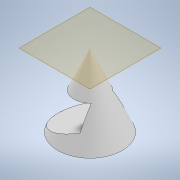
# Autodesk Inventor part: Деталь2Инди
Saved by Autodesk Inventor 2021.1 (Build 251245010, 245A)
## iProperties
Created: 2023-10-12
Part Number: Деталь2Инди
Material: Типовые
Document SubType Name: Modeling
Designer: Lenovo
Density: 1 g/cm^3
Appearance: По умолчанию
Author: Lenovo
Autodesk Inventor part; units mm, degrees
ref_plane "YZ Plane" through (0, 0, 0) normal (1, 0, 0) x (0, 1, 0)
ref_plane "XY Plane" through (0, 0, 0) normal (0, 0, 1) x (1, 0, 0)
sketch "Эскиз1" plane through (0, 0, 0) normal (0, 1, 0) x (-1, 0, 0)
  circle A0 centre (0, 0) radius 40
  dimension "d0" = 80
  constraints: 1 centre point, 1 coincident
  measures "d0" diameter of A0
ref_plane "РабПлоскость1" through (0, 90, 0) normal (0, 1, 0) x (-1, 0, 0)
sketch "Эскиз3" plane through (0, 90, 0) normal (0, 1, 0) x (-1, 0, 0)
  point P0 (0, 0)
  point P1 (0, 0)
loft "Лофт1" add profiles "Эскиз1" section 1 point at (0, 90, 0)
sketch "Эскиз4" plane through (0, 0, 0) normal (0, 0, 1) x (1, 0, 0)
  line L0 (0, 0) -> (15, 0)
  line L1 (40, 0) -> (-40, 0) projected
  line L2 (15, 20) -> (-40, 0)
  line L3 (15, 20) -> (15, 45)
  line L4 (15, 45) -> (-19.9727, 45.0615)
  line L5 (-19.9727, 45.0615) -> (-40, 0)
  line L6 (-40, 0) -> (0, 90) projected
  dimension "d6" = 15
  dimension "d8" = 25
  constraints: 10 end point, 1 collinear, 1 point on line, 1 vertical
  measures "d6" distance of L0.start L0.end
  measures "d8" distance of L2.start L3.end
extrude "Выдавливание1" cut sketch "Эскиз4" along normal mid plane 100
